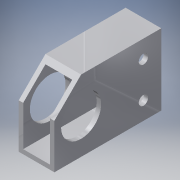
# Autodesk Inventor part: flywheelsupport2
Saved by Autodesk Inventor 2016 (Build 200138000, 138)
## iProperties
Created: 2016-01-29
Part Number: flywheelsupport2
Material: Aluminum 6061
Document SubType Name: Modeling
Designer: zachary
Density: 2.7 g/cm^3
Appearance: Aluminum - Flat
Mass: 27.5176 g
Surface Area: 188.562 cm^2
Volume: 27.5176 cm^3
Author: zachary
Autodesk Inventor part; units mm, degrees
ref_plane "YZ Plane" through (0, 0, 0) normal (1, 0, 0) x (0, 1, 0)
ref_plane "XZ Plane" through (0, 0, 0) normal (0, 1, 0) x (-1, 0, 0)
ref_plane "XY Plane" through (0, 0, 0) normal (0, 0, 1) x (1, 0, 0)
sketch "Sketch1" plane through (0, 0, 0) normal (0, 0, 1) x (1, 0, 0)
  line L0 (0, 0) -> (25.4, 0)
  line L1 (25.4, 0) -> (25.4, -50.8)
  line L2 (25.4, -50.8) -> (0, -50.8)
  line L3 (0, -50.8) -> (0, 0)
  line L4 (22.225, -3.175) -> (3.175, -3.175)
  line L5 (3.175, -3.175) -> (3.175, -47.625)
  line L6 (3.175, -47.625) -> (22.225, -47.625)
  line L7 (22.225, -47.625) -> (22.225, -3.175)
  dimension "d0" = 25.4
  dimension "d1" = 50.8
  dimension "d2" = 3.175
  dimension "d3" = 3.175
  dimension "d4" = 3.175
  dimension "d5" = 3.175
  constraints: 16 end point, 4 parallel, 2 horizontal, 2 perpendicular
  measures "d0" distance between parallel lines of L3 L1
  measures "d1" distance between parallel lines of L0 L2
  measures "d2" distance between parallel lines of L1 L7
  measures "d3" distance between parallel lines of L2 L6
  measures "d4" distance between parallel lines of L3 L5
  measures "d5" distance between parallel lines of L0 L4
extrude "Extrusion1" add sketch "Sketch1" along normal blind 76.2
sketch "Sketch2" plane through (0, -50.8, 0) normal (-1, 0, 0) x (0, 0, 1)
  circle A0 centre (57.15, 25.4) radius 14.2875
  line L0 (76.2, 50.8) -> (76.2, 0) projected
  line L1 (0, 50.8) -> (76.2, 50.8) projected
  dimension "d8" = 28.575
  dimension "d9" = 19.05
  dimension "d10" = 25.4
  constraints: 1 centre point
  measures "d8" diameter of A0
  measures "d9" distance from line of L0 A0.centre
  measures "d10" distance from line of L1 A0.centre
extrude "Extrusion2" cut sketch "Sketch2" against normal through all
sketch "Sketch3" plane through (0, -50.8, 0) normal (-1, 0, 0) x (0, 0, 1)
  line L0 (76.2, 47.625) -> (76.2, 3.175) projected
  line L1 (76.2, 31.75) -> (57.15, 50.8)
  line L2 (0, 50.8) -> (76.2, 50.8) projected
  line L3 (76.2, 0) -> (76.2, 50.8) projected
  line L4 (57.15, 50.8) -> (76.2, 50.8)
  line L5 (76.2, 50.8) -> (76.2, 31.75)
  dimension "d13" = 135
  dimension "d14" = 19.05
  constraints: 6 end point, 2 point on line, 1 collinear, 1 horizontal
  measures "d13" angle of L0 L1
  measures "d14" horizontal distance of L1.start L1.end
extrude "Extrusion3" cut sketch "Sketch3" against normal through all
sketch "Sketch4" plane through (0, -50.8, 0) normal (-1, 0, 0) x (0, 0, 1)
  circle A0 centre (12.7, 12.7) radius 3.3734
  circle A1 centre (12.7, 38.1) radius 3.3734
  line L0 (0, 50.8) -> (57.15, 50.8) projected
  line L1 (0, 0) -> (0, 50.8) projected
  dimension "d17" = 6.7469
  dimension "d18" = 12.7
  dimension "d19" = 38.1
  dimension "d20" = 12.7
  dimension "d21" = 12.7
  constraints: 2 centre point, 1 equal radius
  measures "d17" diameter of A0
  measures "d18" distance from line of L0 A1.centre
  measures "d19" distance from line of L0 A0.centre
  measures "d20" distance from line of L1 A0.centre
  measures "d21" distance from line of L1 A1.centre
extrude "Extrusion4" cut sketch "Sketch4" against normal blind 25.4
body "Solid1"
